Autodesk Inventor part; units mm, degrees
(part 3 of 5)
  arc A1149 (8.6341, 10.3239) -> (7.2074, 10.3304) centre (7.8644, -2.208) ccw
  arc A1150 (10.0591, 10.155) -> (8.6341, 10.3239) centre (7.8573, -2.3245) ccw
  arc A1151 (11.2931, 9.8332) -> (10.0591, 10.155) centre (8.6807, 2.3424) ccw
  arc A1152 (-14.2689, 7.2702) -> (-15.0029, 6.7254) centre (-13.5906, 5.5896) ccw
  arc A1153 (-15.0029, 6.7254) -> (-15.3966, 5.8804) centre (-13.4832, 5.5032) ccw
  arc A1154 (-15.3966, 5.8804) -> (-15.5635, 4.3135) centre (-6.6517, 4.1565) ccw
  arc A1155 (-15.5635, 4.3135) -> (-15.5968, 0.5339) centre (198.9705, 0.534) ccw
  arc A1156 (-15.5968, 0.5339) -> (-15.5855, -2.9927) centre (534.7574, 0.5336) ccw
  arc A1157 (-15.5855, -2.9927) -> (-15.5199, -4.2476) centre (-1.8593, -2.9048) ccw
  arc A1158 (-15.5199, -4.2476) -> (-15.3495, -4.9618) centre (-12.8301, -3.9832) ccw
  arc A1159 (-15.3495, -4.9618) -> (-14.9991, -5.5461) centre (-13.4693, -4.2315) ccw
  arc A1160 (-14.9991, -5.5461) -> (-14.5333, -5.9588) centre (-13.256, -4.0482) ccw
  arc A1161 (-14.5333, -5.9588) -> (-14.0306, -6.1641) centre (-13.7802, -4.8324) ccw
  arc A1162 (-14.0306, -6.1641) -> (-13.1923, -6.2566) centre (-13.0028, -0.6964) ccw
  arc A1163 (-13.1923, -6.2566) -> (-10.8659, -6.323) centre (-6.0064, 204.5863) ccw
  arc A1164 (-10.8659, -6.323) -> (-8.1681, -6.35) centre (-8.4856, 96.9906) ccw
  arc A1165 (-8.1681, -6.35) -> (-6.6957, -6.2434) centre (-8.2009, 4.3293) ccw
  arc A1166 (-6.6957, -6.2434) -> (-5.7509, -5.9784) centre (-7.221, -2.5536) ccw
  arc A1167 (-5.7509, -5.9784) -> (-5.034, -5.4928) centre (-6.6553, -3.8715) ccw
  arc A1168 (-5.034, -5.4928) -> (-4.687, -4.9742) centre (-6.1681, -4.3587) ccw
  arc A1169 (-4.687, -4.9742) -> (-4.518, -4.3054) centre (-6.8723, -4.066) ccw
  arc A1170 (-4.518, -4.3054) -> (-4.453, -3.1016) centre (-17.1608, -3.0197) ccw
  arc A1171 (-4.453, -3.1016) -> (-4.442, 0.3284) centre (-536.7191, 0.3287) ccw
  arc A1172 (-4.442, 0.3284) -> (-4.4832, 4.1346) centre (-180.1506, 0.3283) ccw
  arc A1173 (-4.4832, 4.1346) -> (-4.6809, 5.7903) centre (-13.0751, 3.9485) ccw
  arc A1174 (-4.6809, 5.7903) -> (-5.1333, 6.6851) centre (-6.6435, 5.3596) ccw
  arc A1175 (-5.1333, 6.6851) -> (-5.9587, 7.2413) centre (-6.6019, 5.3961) ccw
  arc A1176 (-5.9587, 7.2413) -> (-7.0837, 7.4475) centre (-7.1851, 3.7233) ccw
  arc A1177 (-7.0837, 7.4475) -> (-10.1664, 7.4949) centre (-10.6188, -122.3153) ccw
  arc A1178 (-10.1664, 7.4949) -> (-13.2748, 7.4725) centre (-10.6734, -137.9503) ccw
  arc A1179 (-13.2748, 7.4725) -> (-14.2689, 7.2702) centre (-13.2249, 4.6832) ccw
  arc A1180 (-14.7169, 5.5669) -> (-14.1838, 6.0865) centre (-34.7338, 26.6365) ccw
  arc A1181 (-14.9423, 5.4172) -> (-14.7169, 5.5669) centre (-15.2572, 6.1357) ccw
  arc A1182 (-15.0561, 5.4626) -> (-14.9423, 5.4172) centre (-14.9769, 5.496) ccw
  arc A1183 (-15.101, 5.6846) -> (-15.0561, 5.4626) centre (-14.5294, 5.6846) ccw
  arc A1184 (-15.0074, 6.0856) -> (-15.101, 5.6846) centre (-14.1956, 5.6846) ccw
  arc A1185 (-14.73, 6.4972) -> (-15.0074, 6.0856) centre (-13.3432, 5.2635) ccw
  arc A1186 (-14.3269, 6.8498) -> (-14.73, 6.4972) centre (-13.1262, 5.0705) ccw
  arc A1187 (-13.8616, 7.0779) -> (-14.3269, 6.8498) centre (-13.2722, 5.2869) ccw
  arc A1188 (-13.5072, 7.1356) -> (-13.8616, 7.0779) centre (-13.5016, 5.9839) ccw
  arc A1189 (-13.4174, 7.0127) -> (-13.5072, 7.1356) centre (-13.5067, 7.0417) ccw
  arc A1190 (-13.6008, 6.6974) -> (-13.4174, 7.0127) centre (-14.2405, 7.2802) ccw
  arc A1191 (-14.1838, 6.0865) -> (-13.6008, 6.6974) centre (-27.0342, 18.9369) ccw
  arc A1192 (-5.369, 6.261) -> (-5.3902, 6.5814) centre (-5.5632, 6.409) ccw
  arc A1193 (-6.1138, 5.3522) -> (-5.369, 6.261) centre (-18.7203, 16.4429) ccw
  arc A1194 (-7.4344, 3.9305) -> (-6.1138, 5.3522) centre (-33.0415, 29.0421) ccw
  arc A1195 (-10.0244, 1.3139) -> (-7.4344, 3.9305) centre (-290.0893, 281.1159) ccw
  arc A1196 (-11.9319, -0.585) -> (-10.0244, 1.3139) centre (-356.2197, 347.1842) ccw
  arc A1197 (-13.5616, -2.1839) -> (-11.9319, -0.585) centre (-190.9648, 180.2579) ccw
  arc A1198 (-15.0178, -3.5983) -> (-13.5616, -2.1839) centre (-1246.2884, 1265.5516) ccw
  arc A1199 (-15.1177, -3.6388) -> (-15.0178, -3.5983) centre (-15.1177, -3.4953) ccw
  arc A1200 (-15.1687, -3.5954) -> (-15.1177, -3.6388) centre (-15.1177, -3.5871) ccw
  arc A1201 (-15.1891, -3.4021) -> (-15.1687, -3.5954) centre (-13.4719, -3.3194) ccw
  arc A1202 (-15.1869, -3.1421) -> (-15.1891, -3.4021) centre (-12.8846, -3.2911) ccw
  arc A1203 (-15.1565, -2.8332) -> (-15.1869, -3.1421) centre (-10.5477, -3.4424) ccw
  arc A1204 (-14.9222, -2.233) -> (-15.1565, -2.8332) centre (-13.8179, -3.0101) ccw
  arc A1205 (-14.2117, -1.3211) -> (-14.9222, -2.233) centre (-5.195, -9.0783) ccw
  arc A1206 (-12.9707, 0.0372) -> (-14.2117, -1.3211) centre (9.1494, -21.4189) ccw
  arc A1207 (-10.6781, 2.3724) -> (-12.9707, 0.0372) centre (182.1892, -189.2648) ccw
  arc A1208 (-10.6781, 2.3724) -> (-9.019, 4.0601) centre (-168.3412, 159.0297) ccw
  arc A1209 (-9.019, 4.0601) -> (-7.6634, 5.4799) centre (-84.9047, 77.8727) ccw
  arc A1210 (-7.6634, 5.4799) -> (-6.5236, 6.7019) centre (-257.9199, 240.0277) ccw
  arc A1211 (-6.5236, 6.7019) -> (-6.5544, 6.7724) centre (-6.5544, 6.7304) ccw
  arc A1212 (-6.5544, 6.7724) -> (-6.7207, 6.7067) centre (-6.5544, 6.5289) ccw
  arc A1213 (-6.7207, 6.7067) -> (-7.9294, 5.5709) centre (238.0969, -255.0416) ccw
  arc A1214 (-7.9294, 5.5709) -> (-9.3033, 4.2502) centre (64.3345, -70.9771) ccw
  arc A1215 (-9.3033, 4.2502) -> (-10.887, 2.6823) centre (127.8746, -135.8883) ccw
  arc A1216 (-12.4629, 1.1142) -> (-10.887, 2.6823) centre (-257.9204, 249.3758) ccw
  arc A1217 (-13.8124, -0.2064) -> (-12.4629, 1.1142) centre (-140.6508, 130.7665) ccw
  arc A1218 (-15.0152, -1.3694) -> (-13.8124, -0.2064) centre (-777.5444, 788.4217) ccw
  arc A1219 (-15.1104, -1.4078) -> (-15.0152, -1.3694) centre (-15.1104, -1.2708) ccw
  arc A1220 (-15.1598, -1.3649) -> (-15.1104, -1.4078) centre (-15.1104, -1.3579) ccw
  arc A1221 (-15.1793, -1.1574) -> (-15.1598, -1.3649) centre (-12.9724, -1.0553) ccw
  arc A1222 (-15.178, -0.8822) -> (-15.1793, -1.1574) centre (-12.4811, -1.0326) ccw
  arc A1223 (-15.1498, -0.5554) -> (-15.178, -0.8822) centre (-9.7652, -1.184) ccw
  arc A1224 (-14.9553, 0.0294) -> (-15.1498, -0.5554) centre (-13.6453, -0.731) ccw
  arc A1225 (-14.4687, 0.7308) -> (-14.9553, 0.0294) centre (-10.3735, -2.6302) ccw
  arc A1226 (-13.5735, 1.7298) -> (-14.4687, 0.7308) centre (-2.5197, -9.0758) ccw
  arc A1227 (-11.8574, 3.4563) -> (-13.5735, 1.7298) centre (90.964, -100.4609) ccw
  arc A1228 (-11.8574, 3.4563) -> (-10.6423, 4.6769) centre (-91.9133, 84.3654) ccw
  arc A1229 (-10.6423, 4.6769) -> (-9.64, 5.7252) centre (-51.7109, 44.9459) ccw
  arc A1230 (-9.64, 5.7252) -> (-8.7905, 6.6422) centre (-153.1351, 139.4989) ccw
  arc A1231 (-8.7905, 6.6422) -> (-8.7926, 6.7438) centre (-8.8445, 6.6919) ccw
  arc A1232 (-8.7926, 6.7438) -> (-8.8943, 6.7463) centre (-8.8448, 6.6916) ccw
  arc A1233 (-8.8943, 6.7463) -> (-9.7737, 5.9459) centre (105.081, -119.365) ccw
  arc A1234 (-9.7737, 5.9459) -> (-10.7808, 4.998) centre (25.5758, -32.6218) ccw
  arc A1235 (-10.7808, 4.998) -> (-11.9525, 3.8475) centre (61.1169, -69.3977) ccw
  arc A1236 (-13.1243, 2.6881) -> (-11.9525, 3.8475) centre (-154.213, 146.4505) ccw
  arc A1237 (-14.1326, 1.7116) -> (-13.1243, 2.6881) centre (-87.5839, 78.5589) ccw
  arc A1238 (-15.0266, 0.8592) -> (-14.1326, 1.7116) centre (-358.2866, 361.7781) ccw
  arc A1239 (-15.1168, 0.8231) -> (-15.0266, 0.8592) centre (-15.1168, 0.954) ccw
  arc A1240 (-15.164, 0.8649) -> (-15.1168, 0.8231) centre (-15.1168, 0.8707) ccw
  arc A1241 (-15.1808, 1.077) -> (-15.164, 0.8649) centre (-12.669, 1.169) ccw
  arc A1242 (-15.1776, 1.3559) -> (-15.1808, 1.077) centre (-12.2736, 1.1835) ccw
  arc A1243 (-15.1485, 1.6872) -> (-15.1776, 1.3559) centre (-9.3449, 1.0097) ccw
  arc A1244 (-14.9951, 2.2222) -> (-15.1485, 1.6872) centre (-13.445, 1.4884) ccw
  arc A1245 (-14.6569, 2.7815) -> (-14.9951, 2.2222) centre (-12.0877, 0.8459) ccw
  arc A1246 (-14.0493, 3.4933) -> (-14.6569, 2.7815) centre (-8.5071, -1.8518) ccw
  arc A1247 (-12.9686, 4.5806) -> (-14.0493, 3.4933) centre (22.4806, -31.7374) ccw
  arc A1248 (-12.9686, 4.5806) -> (-12.1808, 5.368) centre (-45.7482, 38.1635) ccw
  arc A1249 (-12.1808, 5.368) -> (-11.5385, 6.0519) centre (-29.1598, 21.9566) ccw
  arc A1250 (-11.5385, 6.0519) -> (-11.0163, 6.6395) centre (-49.2283, 40.0701) ccw
  arc A1251 (-11.0163, 6.6395) -> (-11.0197, 6.7398) centre (-11.0716, 6.6879) ccw
  arc A1252 (-11.0197, 6.7398) -> (-11.1204, 6.7441) centre (-11.0724, 6.6871) ccw
  arc A1253 (-11.1204, 6.7441) -> (-11.6919, 6.2547) centre (17.8083, -27.6153) ccw
  arc A1254 (-11.6919, 6.2547) -> (-12.3585, 5.6496) centre (2.6791, -10.245) ccw
  arc A1255 (-12.3585, 5.6496) -> (-13.1254, 4.9058) centre (17.2995, -25.6985) ccw
  line L70 (-13.1254, 4.9058) -> (-15.101, 2.9418)
  line L71 (-15.101, 2.9418) -> (-15.101, 3.8604)
  arc A1256 (-15.0485, 4.3869) -> (-15.101, 3.8604) centre (-12.434, 3.8604) ccw
  arc A1257 (-14.8904, 4.8048) -> (-15.0485, 4.3869) centre (-13.698, 4.115) ccw
  arc A1258 (-14.5681, 5.2353) -> (-14.8904, 4.8048) centre (-12.9172, 3.6633) ccw
  arc A1259 (-13.9571, 5.8377) -> (-14.5681, 5.2353) centre (-4.7269, -4.1359) ccw
  arc A1260 (-13.4501, 6.2649) -> (-13.9571, 5.8377) centre (-9.1213, 0.6123) ccw
  arc A1261 (-12.9184, 6.6311) -> (-13.4501, 6.2649) centre (-9.5568, 1.1811) ccw
  arc A1262 (-12.4232, 6.9008) -> (-12.9184, 6.6311) centre (-10.167, 2.1703) ccw
  arc A1263 (-12.0399, 7.0202) -> (-12.4232, 6.9008) centre (-11.817, 5.6299) ccw
  arc A1264 (-10.6511, 7.1146) -> (-12.0399, 7.0202) centre (-10.8287, -0.537) ccw
  arc A1265 (-8.3195, 7.0107) -> (-10.6511, 7.1146) centre (-11.9196, -47.5415) ccw
  arc A1266 (-5.9123, 6.8255) -> (-8.3195, 7.0107) centre (-15.6325, -103.8039) ccw
  arc A1267 (-5.3902, 6.5814) -> (-5.9123, 6.8255) centre (-5.9859, 5.9877) ccw
  arc A1268 (-11.5429, -2.4135) -> (-9.689, -0.5817) centre (-151.916, 141.5052) ccw
  arc A1269 (-13.1444, -3.943) -> (-11.5429, -2.4135) centre (-85.0076, 72.9068) ccw
  arc A1270 (-14.555, -5.2556) -> (-13.1444, -3.943) centre (-278.0551, 279.3503) ccw
  arc A1271 (-14.7274, -5.2932) -> (-14.555, -5.2556) centre (-14.6731, -5.128) ccw
  arc A1272 (-14.8283, -5.2275) -> (-14.7274, -5.2932) centre (-14.6542, -5.0704) ccw
  arc A1273 (-14.9247, -5.0944) -> (-14.8283, -5.2275) centre (-14.2593, -4.7138) ccw
  arc A1274 (-15.0027, -4.9212) -> (-14.9247, -5.0944) centre (-14.0688, -4.6049) ccw
  arc A1275 (-15.0486, -4.7317) -> (-15.0027, -4.9212) centre (-13.9673, -4.5705) ccw
  arc A1276 (-14.9401, -4.3504) -> (-15.0486, -4.7317) centre (-14.5734, -4.6608) ccw
  arc A1277 (-13.9274, -3.1917) -> (-14.9401, -4.3504) centre (22.1213, -35.7196) ccw
  arc A1278 (-12.4307, -1.5992) -> (-13.9274, -3.1917) centre (26.1037, -39.313) ccw
  arc A1279 (-10.0909, 0.7626) -> (-12.4307, -1.5992) centre (182.391, -192.2721) ccw
  arc A1280 (-6.8029, 4.0259) -> (-10.0909, 0.7626) centre (688.2331, -699.5646) ccw
  arc A1281 (-5.7215, 5.0044) -> (-6.8029, 4.0259) centre (4.9025, -7.8236) ccw
  arc A1282 (-5.2387, 5.2053) -> (-5.7215, 5.0044) centre (-5.152, 4.3167) ccw
  arc A1283 (-4.9809, 4.9946) -> (-5.2387, 5.2053) centre (-5.2158, 4.9704) ccw
  arc A1284 (-5.1077, 4.3788) -> (-4.9809, 4.9946) centre (-6.0196, 4.8875) ccw
  arc A1285 (-5.6506, 3.5937) -> (-5.1077, 4.3788) centre (-9.4491, 6.8007) ccw
  arc A1286 (-6.807, 2.3253) -> (-5.6506, 3.5937) centre (-22.8922, 18.1506) ccw
  arc A1287 (-9.689, -0.5817) -> (-6.807, 2.3253) centre (-388.1467, 377.5026) ccw
  arc A1288 (-11.1643, -4.2674) -> (-8.8203, -1.944) centre (-236.5359, 225.4382) ccw
  arc A1289 (-12.2567, -5.2477) -> (-11.1643, -4.2674) centre (-22.7028, 7.4931) ccw
  arc A1290 (-12.9748, -5.7175) -> (-12.2567, -5.2477) centre (-14.7932, -2.154) ccw
  arc A1291 (-13.6083, -5.8698) -> (-12.9748, -5.7175) centre (-13.6083, -4.4759) ccw
  arc A1292 (-13.8587, -5.6594) -> (-13.6083, -5.8698) centre (-13.6083, -5.6156) ccw
  arc A1293 (-13.7543, -5.259) -> (-13.8587, -5.6594) centre (-13.368, -5.5736) ccw
  arc A1294 (-12.8767, -4.2816) -> (-13.7543, -5.259) centre (-3.2069, -13.8466) ccw
  arc A1295 (-9.769, -1.1543) -> (-12.8767, -4.2816) centre (670.3181, -680.0673) ccw
  arc A1296 (-6.6738, 1.9312) -> (-9.769, -1.1543) centre (626.6559, -636.4816) ccw
  arc A1297 (-5.6713, 2.8358) -> (-6.6738, 1.9312) centre (3.3784, -8.2017) ccw
  arc A1298 (-5.2271, 2.9942) -> (-5.6713, 2.8358) centre (-5.2284, 2.2957) ccw
  arc A1299 (-4.981, 2.7715) -> (-5.2271, 2.9942) centre (-5.2276, 2.7463) ccw
  arc A1300 (-5.0849, 2.1811) -> (-4.981, 2.7715) centre (-6.0751, 2.6597) ccw
  arc A1301 (-5.5218, 1.4946) -> (-5.0849, 2.1811) centre (-8.235, 3.7036) ccw
  arc A1302 (-6.4749, 0.4278) -> (-5.5218, 1.4946) centre (-17.6327, 11.3551) ccw
  arc A1303 (-8.8203, -1.944) -> (-6.4749, 0.4278) centre (-252.0588, 240.9382) ccw
  arc A1304 (-4.9861, -3.5076) -> (-4.9712, -1.7177) centre (-109.4566, -1.7426) ccw
  arc A1305 (-5.0546, -4.3559) -> (-4.9861, -3.5076) centre (-11.6752, -3.3946) ccw
  arc A1306 (-5.2075, -4.8827) -> (-5.0546, -4.3559) centre (-7.0219, -4.0703) ccw
  arc A1307 (-5.4931, -5.312) -> (-5.2075, -4.8827) centre (-6.6319, -4.2449) ccw
  arc A1308 (-5.7778, -5.5571) -> (-5.4931, -5.312) centre (-6.7749, -4.1109) ccw
  arc A1309 (-6.1037, -5.7315) -> (-5.7778, -5.5571) centre (-6.7139, -4.1994) ccw
  arc A1310 (-6.4748, -5.8351) -> (-6.1037, -5.7315) centre (-6.772, -4.0536) ccw
  arc A1311 (-6.8936, -5.8698) -> (-6.4748, -5.8351) centre (-6.8936, -3.3244) ccw
  line L72 (-6.8936, -5.8698) -> (-7.7715, -5.8698)
  line L73 (-7.7715, -5.8698) -> (-6.4785, -4.5606)
  arc A1312 (-6.4785, -4.5606) -> (-5.9832, -4.042) centre (-21.8725, 10.6422) ccw
  arc A1313 (-5.9832, -4.042) -> (-5.5654, -3.5675) centre (-15.6012, 4.8466) ccw
  arc A1314 (-5.5654, -3.5675) -> (-5.235, -3.1609) centre (-18.6733, 7.4222) ccw
  arc A1315 (-5.235, -3.1609) -> (-5.1856, -3.0184) centre (-5.4159, -3.0184) ccw
  arc A1316 (-5.1856, -3.0184) -> (-5.2482, -2.9874) centre (-5.2246, -3.0184) ccw
  arc A1317 (-5.2482, -2.9874) -> (-5.6407, -3.2991) centre (2.2216, -12.7978) ccw
  arc A1318 (-5.6407, -3.2991) -> (-6.1404, -3.7359) centre (2.195, -12.7657) ccw
  arc A1319 (-6.1404, -3.7359) -> (-6.7349, -4.3008) centre (13.1199, -24.6008) ccw
  arc A1320 (-7.4945, -5.0061) -> (-6.7349, -4.3008) centre (-20.6865, 9.9637) ccw
  arc A1321 (-8.1102, -5.4868) -> (-7.4945, -5.0061) centre (-11.8413, -0.0736) ccw
  arc A1322 (-8.6313, -5.7878) -> (-8.1102, -5.4868) centre (-10.2556, -2.3741) ccw
  arc A1323 (-9.0898, -5.9239) -> (-8.6313, -5.7878) centre (-9.2946, -4.3938) ccw
  arc A1324 (-9.3987, -5.9546) -> (-9.0898, -5.9239) centre (-9.696, -1.3946) ccw
  arc A1325 (-9.6588, -5.9567) -> (-9.3987, -5.9546) centre (-9.5462, -3.6923) ccw
  arc A1326 (-9.8515, -5.9358) -> (-9.6588, -5.9567) centre (-9.5762, -4.295) ccw
  arc A1327 (-9.8954, -5.8839) -> (-9.8515, -5.9358) centre (-9.8428, -5.8839) ccw
  arc A1328 (-9.8564, -5.785) -> (-9.8954, -5.8839) centre (-9.7507, -5.8839) ccw
  arc A1329 (-9.2037, -5.0906) -> (-9.8564, -5.785) centre (130.4768, -137.0342) ccw
  arc A1330 (-8.4432, -4.3005) -> (-9.2037, -5.0906) centre (33.2795, -45.2206) ccw
  arc A1331 (-7.5405, -3.3909) -> (-8.4432, -4.3005) centre (69.1214, -80.3729) ccw
  arc A1332 (-7.5405, -3.3909) -> (-6.638, -2.4741) centre (-53.3898, 42.6497) ccw
  arc A1333 (-6.638, -2.4741) -> (-5.8774, -1.6617) centre (-32.9016, 22.8749) ccw
  arc A1334 (-5.8774, -1.6617) -> (-5.2464, -0.9577) centre (-60.4698, 47.9053) ccw
  arc A1335 (-5.2464, -0.9577) -> (-5.1856, -0.7972) centre (-5.4278, -0.7972) ccw
  arc A1336 (-5.1856, -0.7972) -> (-5.2548, -0.7657) centre (-5.2274, -0.7972) ccw
  arc A1337 (-5.2548, -0.7657) -> (-5.9684, -1.3956) centre (38.7824, -51.3747) ccw
  arc A1338 (-5.9684, -1.3956) -> (-6.8281, -2.1903) centre (18.6502, -28.8905) ccw
  arc A1339 (-6.8281, -2.1903) -> (-7.8504, -3.1832) centre (48.7205, -60.4029) ccw
  arc A1340 (-9.2202, -4.5061) -> (-7.8504, -3.1832) centre (-64.9801, 54.6016) ccw
  arc A1341 (-10.1256, -5.2882) -> (-9.2202, -4.5061) centre (-18.5892, 5.4254) ccw
  arc A1342 (-10.7924, -5.7434) -> (-10.1256, -5.2882) centre (-13.7225, -0.7351) ccw
  arc A1343 (-11.3208, -5.9248) -> (-10.7924, -5.7434) centre (-11.5071, -4.5219) ccw
  arc A1344 (-11.6297, -5.9557) -> (-11.3208, -5.9248) centre (-11.957, -1.1342) ccw
  arc A1345 (-11.8897, -5.9593) -> (-11.6297, -5.9557) centre (-11.792, -3.5647) ccw
  arc A1346 (-12.084, -5.941) -> (-11.8897, -5.9593) centre (-11.8145, -4.1167) ccw
  arc A1347 (-12.1264, -5.8919) -> (-12.084, -5.941) centre (-12.0768, -5.8919) ccw
  arc A1348 (-12.0627, -5.7363) -> (-12.1264, -5.8919) centre (-11.9047, -5.8919) ccw
  arc A1349 (-8.6188, -2.2402) -> (-12.0627, -5.7363) centre (7273.2468, -7178.6542) ccw
  arc A1350 (-5.1724, 1.2552) -> (-8.6188, -2.2402) centre (7336.2909, -7240.7819) ccw
  arc A1351 (-5.02, 1.3189) -> (-5.1724, 1.2552) centre (-5.02, 1.1048) ccw
  arc A1352 (-5.0003, 1.2995) -> (-5.02, 1.3189) centre (-5.02, 1.2992) ccw
  arc A1353 (-4.9858, 0.4269) -> (-5.0003, 1.2995) centre (-888.2077, -13.7685) ccw
  arc A1354 (-4.9749, -0.5533) -> (-4.9858, 0.4269) centre (-103.9909, -1.1645) ccw
  arc A1355 (-4.9712, -1.7177) -> (-4.9749, -0.5533) centre (-201.1281, -1.7643) ccw
  arc A1356 (-47.5872, 6.4838) -> (-47.7919, 6.3363) centre (-38.3913, -6.4958) ccw
  arc A1357 (-47.7919, 6.3363) -> (-47.8023, 6.3017) centre (-47.7742, 6.3122) ccw
  arc A1358 (-47.8023, 6.3017) -> (-47.7727, 6.287) centre (-47.7796, 6.3101) ccw
  arc A1359 (-47.7727, 6.287) -> (-47.5404, 6.3585) centre (-51.7296, 19.5602) ccw
  arc A1360 (-47.3446, 6.3797) -> (-47.5404, 6.3585) centre (-47.39, 5.8845) ccw
  arc A1361 (-47.088, 6.333) -> (-47.3446, 6.3797) centre (-47.4787, 4.9144) ccw
  arc A1362 (-46.816, 6.2331) -> (-47.088, 6.333) centre (-47.5516, 4.6499) ccw
  arc A1363 (-46.5697, 6.0911) -> (-46.816, 6.2331) centre (-47.4973, 4.7667) ccw
  arc A1364 (-46.5697, 6.0911) -> (-46.3623, 5.9563) centre (-44.5142, 9.0258) ccw
  arc A1365 (-46.3623, 5.9563) -> (-46.223, 5.8964) centre (-46.0747, 6.434) ccw
  arc A1366 (-46.223, 5.8964) -> (-46.1771, 5.9196) centre (-46.2128, 5.9333) ccw
  arc A1367 (-46.1771, 5.9196) -> (-46.1832, 5.9845) centre (-46.2457, 5.9459) ccw
  arc A1368 (-46.1832, 5.9845) -> (-46.4751, 6.3144) centre (-47.2857, 5.3031) ccw
  arc A1369 (-46.4751, 6.3144) -> (-46.8627, 6.5306) centre (-47.31, 5.2728) ccw
  arc A1370 (-46.8627, 6.5306) -> (-47.2615, 6.5931) centre (-47.2279, 5.5037) ccw
  arc A1371 (-47.2615, 6.5931) -> (-47.5872, 6.4838) centre (-47.2431, 5.9981) ccw
  arc A1372 (-48.0789, 4.9627) -> (-47.7011, 4.6858) centre (-47.4249, 5.4589) ccw
  arc A1373 (-47.7011, 4.6858) -> (-47.1514, 4.5938) centre (-47.1694, 6.174) ccw
  arc A1374 (-47.1514, 4.5938) -> (-46.6597, 4.7) centre (-47.1657, 5.8505) ccw
  arc A1375 (-46.6597, 4.7) -> (-46.4341, 4.9814) centre (-46.8168, 5.0571) ccw
  arc A1376 (-46.4341, 4.9814) -> (-46.415, 5.0949) centre (-48.4188, 5.3738) ccw
  arc A1377 (-46.415, 5.0949) -> (-46.427, 5.13) centre (-46.4557, 5.1006) ccw
  arc A1378 (-46.427, 5.13) -> (-46.4514, 5.1269) centre (-46.438, 5.1187) ccw
  arc A1379 (-46.4514, 5.1269) -> (-46.4976, 5.0434) centre (-45.5437, 4.5703) ccw
  arc A1380 (-46.736, 4.8493) -> (-46.4976, 5.0434) centre (-46.8301, 5.2083) ccw
  arc A1381 (-47.1922, 4.7987) -> (-46.736, 4.8493) centre (-47.1363, 6.3761) ccw
  arc A1382 (-47.6925, 4.8847) -> (-47.1922, 4.7987) centre (-47.1253, 6.6865) ccw
  arc A1383 (-48.0701, 5.0991) -> (-47.6925, 4.8847) centre (-47.3821, 5.8707) ccw
  arc A1384 (-48.0701, 5.0991) -> (-48.2761, 5.2809) centre (-65.2264, -14.1402) ccw
  arc A1385 (-48.2761, 5.2809) -> (-48.2944, 5.2732) centre (-48.2833, 5.2725) ccw
  arc A1386 (-48.2944, 5.2732) -> (-48.2822, 5.2323) centre (-48.2328, 5.2693) ccw
  arc A1387 (-48.2822, 5.2323) -> (-48.0789, 4.9627) centre (-3.2497, 38.9768) ccw
  arc A1388 (-54.9842, 2.087) -> (-55.6668, 0.9823) centre (-53.2977, 0.2817) ccw
  arc A1389 (-55.6668, 0.9823) -> (-55.6108, -0.2103) centre (-53.9229, 0.4666) ccw
  arc A1390 (-55.6108, -0.2103) -> (-54.8228, -1.1293) centre (-53.8639, 0.4902) ccw
  arc A1391 (-54.8228, -1.1293) -> (-53.5471, -1.4967) centre (-53.4779, 1.142) ccw
  arc A1392 (-53.5471, -1.4967) -> (-52.9687, -1.4805) centre (-53.4075, 3.8295) ccw
  arc A1393 (-52.9687, -1.4805) -> (-52.5723, -1.387) centre (-53.0816, -0.114) ccw
  arc A1394 (-52.5723, -1.387) -> (-52.2428, -1.1875) centre (-53.0105, -0.2916) ccw
  arc A1395 (-52.2428, -1.1875) -> (-51.8873, -0.8327) centre (-54.3957, 1.3249) ccw
  arc A1396 (-51.8873, -0.8327) -> (-51.3873, 0.05) centre (-53.8722, 0.8746) ccw
  arc A1397 (-51.3873, 0.05) -> (-51.3289, 0.9689) centre (-53.107, 0.6207) ccw
  arc A1398 (-51.3289, 0.9689) -> (-51.7297, 1.7992) centre (-53.1132, 0.6195) ccw
  arc A1399 (-51.7297, 1.7992) -> (-52.5266, 2.4318) centre (-53.7404, 0.0846) ccw
  arc A1400 (-52.5266, 2.4318) -> (-53.246, 2.7227) centre (-54.4468, -1.2814) ccw
  arc A1401 (-53.246, 2.7227) -> (-53.8229, 2.7667) centre (-53.6349, 1.426) ccw
  arc A1402 (-53.8229, 2.7667) -> (-54.3672, 2.5657) centre (-53.6335, 1.4164) ccw
  arc A1403 (-54.3672, 2.5657) -> (-54.9842, 2.087) centre (-52.0702, -1.0324) ccw
  arc A1404 (-51.9454, 1.3028) -> (-52.2837, 1.8147) centre (-53.3677, 0.7307) ccw
  arc A1405 (-51.8069, 0.6651) -> (-51.9454, 1.3028) centre (-53.7496, 0.577) ccw
  arc A1406 (-51.8856, -0.0049) -> (-51.8069, 0.6651) centre (-53.8932, 0.5705) ccw
  arc A1407 (-52.1738, -0.609) -> (-51.8856, -0.0049) centre (-53.8334, 0.5534) ccw
  arc A1408 (-52.6738, -1.0129) -> (-52.1738, -0.609) centre (-53.1252, 0.0574) ccw
  arc A1409 (-53.3968, -1.1672) -> (-52.6738, -1.0129) centre (-53.4388, 0.8008) ccw
  arc A1410 (-54.1575, -1.0453) -> (-53.3968, -1.1672) centre (-53.4426, 0.9823) ccw
  arc A1411 (-54.7625, -0.6642) -> (-54.1575, -1.0453) centre (-53.6205, 0.4779) ccw
  arc A1412 (-55.2241, 0.217) -> (-54.7625, -0.6642) centre (-53.5836, 0.5148) ccw
  arc A1413 (-55.1151, 1.2255) -> (-55.2241, 0.217) centre (-53.4623, 0.5368) ccw
  arc A1414 (-54.4754, 2.0144) -> (-55.1151, 1.2255) centre (-53.4567, 0.5345) ccw
  arc A1415 (-53.5231, 2.3104) -> (-54.4754, 2.0144) centre (-53.5231, 0.6309) ccw
  arc A1416 (-53.2004, 2.2743) -> (-53.5231, 2.3104) centre (-53.5231, 0.8503) ccw
  arc A1417 (-52.8518, 2.1658) -> (-53.2004, 2.2743) centre (-53.7128, 0.0131) ccw
  arc A1418 (-52.5288, 2.0058) -> (-52.8518, 2.1658) centre (-53.695, 0.0578) ccw
  arc A1419 (-52.2837, 1.8147) -> (-52.5288, 2.0058) centre (-53.1795, 0.9189) ccw
  arc A1420 (-48.0201, -3.6884) -> (-48.1327, -3.8305) centre (-47.4621, -4.2464) ccw
  arc A1421 (-48.1327, -3.8305) -> (-48.2252, -4.0113) centre (-47.0822, -4.4819) ccw
  arc A1422 (-48.2252, -4.0113) -> (-48.2855, -4.2012) centre (-47.1181, -4.4672) ccw
  arc A1423 (-48.2855, -4.2012) -> (-48.3008, -4.37) centre (-47.666, -4.3423) ccw
  arc A1424 (-48.3008, -4.37) -> (-48.2766, -4.5038) centre (-47.7965, -4.348) ccw
  arc A1425 (-48.2766, -4.5038) -> (-48.223, -4.5245) centre (-48.2414, -4.4924) ccw
  arc A1426 (-48.223, -4.5245) -> (-48.1426, -4.4432) centre (-48.3295, -4.3385) ccw
  arc A1427 (-48.1426, -4.4432) -> (-48.0209, -4.2099) centre (-51.9333, -2.3195) ccw
  arc A1428 (-47.8586, -3.9745) -> (-48.0209, -4.2099) centre (-47.1804, -4.616) ccw
  arc A1429 (-47.6236, -3.783) -> (-47.8586, -3.9745) centre (-47.005, -4.7819) ccw
  arc A1430 (-47.3272, -3.645) -> (-47.6236, -3.783) centre (-46.8972, -4.9559) ccw
  arc A1431 (-46.9842, -3.5678) -> (-47.3272, -3.645) centre (-46.7541, -5.3923) ccw
  line L74 (-46.9842, -3.5678) -> (-46.2105, -3.4702)
  line L75 (-46.2105, -3.4702) -> (-46.9666, -3.4306)
  arc A1432 (-46.9666, -3.4306) -> (-47.2778, -3.4374) centre (-47.0766, -5.5275) ccw
  arc A1433 (-47.2778, -3.4374) -> (-47.5879, -3.4899) centre (-47.0683, -5.6132) ccw
  arc A1434 (-47.5879, -3.4899) -> (-47.8531, -3.5768) centre (-47.1538, -5.264) ccw
  arc A1435 (-47.8531, -3.5768) -> (-48.0201, -3.6884) centre (-47.656, -4.0525) ccw
  arc A1436 (-46.6917, -5.01) -> (-46.8592, -5.1502) centre (-45.3579, -6.7735) ccw
  arc A1437 (-46.8592, -5.1502) -> (-46.9537, -5.2671) centre (-46.5039, -5.5344) ccw
  arc A1438 (-46.9537, -5.2671) -> (-46.9597, -5.3384) centre (-46.8832, -5.309) ccw
  arc A1439 (-46.9597, -5.3384) -> (-46.908, -5.374) centre (-46.908, -5.3185) ccw
  arc A1440 (-46.908, -5.374) -> (-46.7846, -5.3481) centre (-46.908, -5.0676) ccw
  arc A1441 (-46.7846, -5.3481) -> (-46.6302, -5.2648) centre (-47.2239, -4.349) ccw
  arc A1442 (-46.6302, -5.2648) -> (-46.4721, -5.1444) centre (-47.3486, -4.1567) ccw
  arc A1443 (-46.4721, -5.1444) -> (-46.3345, -5.0022) centre (-47.3359, -4.171) ccw
  arc A1444 (-46.3345, -5.0022) -> (-46.1066, -4.7102) centre (-51.1085, -1.0401) ccw
  arc A1445 (-46.1066, -4.7102) -> (-46.1351, -4.6553) centre (-46.1344, -4.6898) ccw
  arc A1446 (-46.1351, -4.6553) -> (-46.2723, -4.7011) centre (-46.1297, -4.8998) ccw
  arc A1447 (-46.2723, -4.7011) -> (-46.6917, -5.01) centre (-34.2808, -21.4187) ccw
  arc A1448 (-48.0696, -5.1261) -> (-47.9091, -5.2181) centre (-47.1309, -3.6735) ccw
  arc A1449 (-47.9091, -5.2181) -> (-47.7342, -5.2958) centre (-47.0192, -3.4519) ccw
  arc A1450 (-47.7342, -5.2958) -> (-47.5707, -5.35) centre (-47.1104, -3.6869) ccw
  arc A1451 (-47.5707, -5.35) -> (-47.4499, -5.3664) centre (-47.4499, -4.9136) ccw
  arc A1452 (-47.4499, -5.3664) -> (-47.3924, -5.3436) centre (-47.4499, -5.2821) ccw
  arc A1453 (-47.3924, -5.3436) -> (-47.3841, -5.2958) centre (-47.4199, -5.3143) ccw
  arc A1454 (-47.3841, -5.2958) -> (-47.4464, -5.2189) centre (-47.6003, -5.4073) ccw
  arc A1455 (-47.4464, -5.2189) -> (-47.5739, -5.1261) centre (-48.3441, -6.318) ccw
  arc A1456 (-47.5739, -5.1261) -> (-47.7344, -5.0341) centre (-48.5126, -6.5787) ccw
  arc A1457 (-47.7344, -5.0341) -> (-47.9093, -4.9564) centre (-48.6243, -6.8003) ccw
  arc A1458 (-47.9093, -4.9564) -> (-48.0728, -4.9022) centre (-48.5332, -6.5653) ccw
  arc A1459 (-48.0728, -4.9022) -> (-48.1936, -4.8858) centre (-48.1936, -5.3386) ccw
  arc A1460 (-48.1936, -4.8858) -> (-48.2512, -4.9085) centre (-48.1936, -4.9701) ccw
  arc A1461 (-48.2512, -4.9085) -> (-48.2594, -4.9564) centre (-48.2237, -4.9379) ccw
  arc A1462 (-48.2594, -4.9564) -> (-48.1971, -5.0333) centre (-48.0432, -4.8448) ccw
  arc A1463 (-48.1971, -5.0333) -> (-48.0696, -5.1261) centre (-47.2994, -3.9342) ccw
  arc A1464 (-28.2732, -5.574) -> (-28.5168, -5.8584) centre (-27.8393, -6.1922) ccw
  arc A1465 (-28.5168, -5.8584) -> (-28.6535, -6.2864) centre (-27.1573, -6.5281) ccw
  arc A1466 (-28.6535, -6.2864) -> (-28.7191, -7.0064) centre (-23.4918, -7.1203) ccw
  arc A1467 (-28.7191, -7.0064) -> (-28.7346, -8.43) centre (36.6219, -8.43) ccw
  line L76 (-28.7346, -8.43) -> (-28.7346, -10.9622)
  line L77 (-28.7346, -10.9622) -> (-27.6117, -12.1853)
  line L78 (-27.6117, -12.1853) -> (-26.4888, -13.4084)
  line L79 (-26.4888, -13.4084) -> (-23.1484, -10.075)
  arc A1468 (-21.3525, -8.3073) -> (-23.1484, -10.075) centre (105.8396, -139.3289) ccw
  arc A1469 (-20.3731, -7.432) -> (-21.3525, -8.3073) centre (-10.2474, -19.7467) ccw
  arc A1470 (-19.7489, -6.9923) -> (-20.3731, -7.432) centre (-17.1151, -11.3943) ccw
  arc A1471 (-19.4042, -6.9963) -> (-19.7489, -6.9923) centre (-19.5799, -7.2748) ccw
  arc A1472 (-19.2503, -7.1087) -> (-19.4042, -6.9963) centre (-20.1555, -8.1874) ccw
  arc A1473 (-19.1214, -7.2355) -> (-19.2503, -7.1087) centre (-19.984, -7.983) ccw
  arc A1474 (-19.0328, -7.3579) -> (-19.1214, -7.2355) centre (-19.7766, -7.8033) ccw
  arc A1475 (-19.0086, -7.4529) -> (-19.0328, -7.3579) centre (-19.1797, -7.4459) ccw
  arc A1476 (-19.0648, -7.5881) -> (-19.0086, -7.4529) centre (-19.2205, -7.4442) ccw
  arc A1477 (-19.9429, -8.5337) -> (-19.0648, -7.5881) centre (-217.3375, 175.6569) ccw
  arc A1478 (-20.9654, -9.61) -> (-19.9429, -8.5337) centre (-80.3638, 47.8456) ccw
  arc A1479 (-22.1776, -10.849) -> (-20.9654, -9.61) centre (-130.9902, 96.8162) ccw
  arc A1480 (-24.0448, -12.7158) -> (-22.1776, -10.849) centre (-194.9979, 160.1492) ccw
  arc A1481 (-24.8728, -13.4507) -> (-24.0448, -12.7158) centre (-31.2632, -5.4166) ccw
  arc A1482 (-25.3484, -13.7097) -> (-24.8728, -13.4507) centre (-25.8516, -12.2202) ccw
  arc A1483 (-25.6528, -13.6133) -> (-25.3484, -13.7097) centre (-25.4348, -13.4538) ccw
  arc A1484 (-25.6528, -13.6133) -> (-25.7858, -13.4611) centre (-26.5955, -14.3026) ccw
  arc A1485 (-25.7858, -13.4611) -> (-25.9253, -13.3598) centre (-26.219, -13.9113) ccw
  arc A1486 (-25.9253, -13.3598) -> (-26.0491, -13.3224) centre (-26.0816, -13.6532) ccw
  arc A1487 (-26.0491, -13.3224) -> (-26.1388, -13.3545) centre (-26.06, -13.4333) ccw
  arc A1488 (-26.1388, -13.3545) -> (-26.1413, -13.6754) centre (-25.977, -13.5162) ccw
  arc A1489 (-26.1413, -13.6754) -> (-24.322, -15.5252) centre (95.7981, 104.4298) ccw
  arc A1490 (-24.322, -15.5252) -> (-22.5035, -17.309) centre (62.9595, 71.6366) ccw
  arc A1491 (-22.5035, -17.309) -> (-21.9787, -17.5203) centre (-21.9787, -16.7628) ccw
  arc A1492 (-21.9787, -17.5203) -> (-21.3796, -17.3874) centre (-21.9787, -16.1034) ccw
  arc A1493 (-21.3796, -17.3874) -> (-18.4307, -15.997) centre (-192.0716, 348.4457) ccw
  arc A1494 (-18.4307, -15.997) -> (-15.5918, -14.6227) centre (-127.4533, 212.8237) ccw
  arc A1495 (-15.5918, -14.6227) -> (-14.7911, -14.0958) centre (-17.2888, -11.172) ccw
  arc A1496 (-14.7911, -14.0958) -> (-14.5875, -13.8415) centre (-15.3556, -13.435) ccw
  arc A1497 (-14.5875, -13.8415) -> (-14.4544, -13.4901) centre (-15.9236, -13.1345) ccw
  arc A1498 (-14.4544, -13.4901) -> (-14.3798, -13.0002) centre (-17.2426, -12.8152) ccw
  arc A1499 (-14.3798, -13.0002) -> (-14.3573, -12.3038) centre (-25.1558, -12.3038) ccw
  arc A1500 (-14.3573, -12.3038) -> (-14.4628, -11.1978) centre (-20.2096, -12.3038) ccw
  arc A1501 (-14.4628, -11.1978) -> (-14.7964, -10.4635) centre (-16.1542, -11.5233) ccw
  arc A1502 (-14.7964, -10.4635) -> (-15.5806, -9.65) centre (-19.0746, -13.8029) ccw
  arc A1503 (-15.5806, -9.65) -> (-17.9814, -7.6611) centre (-147.7014, -166.6845) ccw
  line L80 (-17.9814, -7.6611) -> (-20.7378, -5.4126)
  line L81 (-20.7378, -5.4126) -> (-24.2748, -5.3313)
  arc A1504 (-24.2748, -5.3313) -> (-26.0018, -5.3081) centre (-26.3564, -95.9231) ccw
  arc A1505 (-26.0018, -5.3081) -> (-27.1286, -5.34) centre (-26.0702, -22.7818) ccw
  arc A1506 (-27.1286, -5.34) -> (-27.8876, -5.4197) centre (-26.6035, -13.994) ccw
  arc A1507 (-27.8876, -5.4197) -> (-28.2732, -5.574) centre (-27.7536, -6.3142) ccw
  arc A1508 (-27.4301, -7.1648) -> (-26.9995, -6.7373) centre (-43.5695, 9.5249) ccw
  arc A1509 (-27.8177, -7.5252) -> (-27.4301, -7.1648) centre (-36.7939, 2.5183) ccw
  arc A1510 (-28.1514, -7.8172) -> (-27.8177, -7.5252) centre (-42.127, 8.4855) ccw
  arc A1511 (-28.2476, -7.8528) -> (-28.1514, -7.8172) centre (-28.2476, -7.705) ccw
  arc A1512 (-28.3383, -7.7594) -> (-28.2476, -7.8528) centre (-28.2476, -7.7621) ccw
  arc A1513 (-28.3053, -7.1248) -> (-28.3383, -7.7594) centre (-14.261, -8.172) ccw
  arc A1514 (-28.2286, -6.4607) -> (-28.3053, -7.1248) centre (-20.1054, -7.7362) ccw
  arc A1515 (-28.1043, -5.9317) -> (-28.2286, -6.4607) centre (-24.6431, -7.0237) ccw
  arc A1516 (-27.9974, -5.8058) -> (-28.1043, -5.9317) centre (-27.9012, -5.9958) ccw
  arc A1517 (-27.742, -5.7079) -> (-27.9974, -5.8058) centre (-27.3943, -6.997) ccw
  arc A1518 (-27.3867, -5.643) -> (-27.742, -5.7079) centre (-27.1734, -7.8159) ccw
  arc A1519 (-26.9556, -5.6219) -> (-27.3867, -5.643) centre (-26.9556, -10.0338) ccw
  line L82 (-26.9556, -5.6219) -> (-25.9047, -5.6219)
  line L83 (-25.9047, -5.6219) -> (-26.9995, -6.7373)
  arc A1520 (-26.7603, -8.8361) -> (-25.8984, -7.9438) centre (-102.625, 65.2993) ccw
  arc A1521 (-27.5139, -9.5933) -> (-26.7603, -8.8361) centre (-68.6026, 32.0524) ccw
  arc A1522 (-28.173, -10.2399) -> (-27.5139, -9.5933) centre (-140.9676, 105.3981) ccw
  arc A1523 (-28.2853, -10.2987) -> (-28.173, -10.2399) centre (-28.3273, -10.0818) ccw
  arc A1524 (-28.3434, -10.2582) -> (-28.2853, -10.2987) centre (-28.2947, -10.2502) ccw
  arc A1525 (-28.3636, -10.0489) -> (-28.3434, -10.2582) centre (-26.7633, -10.0001) ccw
  arc A1526 (-28.3553, -9.7563) -> (-28.3636, -10.0489) centre (-25.8742, -9.973) ccw
  arc A1527 (-28.3126, -9.4021) -> (-28.3553, -9.7563) centre (-22.929, -10.2303) ccw
  arc A1528 (-28.1729, -8.8974) -> (-28.3126, -9.4021) centre (-26.1032, -9.742) ccw
  arc A1529 (-27.9035, -8.3618) -> (-28.1729, -8.8974) centre (-24.6395, -10.3392) ccw
  arc A1530 (-27.4891, -7.7661) -> (-27.9035, -8.3618) centre (-22.9808, -11.3441) ccw
  arc A1531 (-26.9029, -7.0752) -> (-27.4891, -7.7661) centre (-16.6609, -16.3601) ccw
  arc A1532 (-26.1619, -6.2949) -> (-26.9029, -7.0752) centre (-9.6253, -22.7381) ccw
  arc A1533 (-25.6856, -5.912) -> (-26.1619, -6.2949) centre (-24.2086, -8.2372) ccw
  arc A1534 (-25.2375, -5.7243) -> (-25.6856, -5.912) centre (-24.9125, -7.129) ccw
  arc A1535 (-24.659, -5.6499) -> (-25.2375, -5.7243) centre (-24.5748, -8.5889) ccw
  line L84 (-24.659, -5.6499) -> (-23.682, -5.6219)
  line L85 (-23.682, -5.6219) -> (-25.8984, -7.9438)
  arc A1536 (-26.3562, -10.5347) -> (-24.4561, -8.6534) centre (-214.1373, 181.0275) ccw
  arc A1537 (-27.1092, -11.1826) -> (-26.3562, -10.5347) centre (-31.7158, -5.0672) ccw
  arc A1538 (-27.5566, -11.3736) -> (-27.1092, -11.1826) centre (-27.72, -10.3718) ccw
  arc A1539 (-27.9142, -11.2583) -> (-27.5566, -11.3736) centre (-27.6229, -10.967) ccw
  arc A1540 (-28.0493, -10.9185) -> (-27.9142, -11.2583) centre (-27.5876, -10.9317) ccw
  arc A1541 (-27.9203, -10.5202) -> (-28.0493, -10.9185) centre (-27.3042, -10.9398) ccw
  arc A1542 (-27.4016, -9.8725) -> (-27.9203, -10.5202) centre (-23.4916, -13.5359) ccw
  arc A1543 (-25.873, -8.2606) -> (-27.4016, -9.8725) centre (107.0624, -135.8561) ccw
  arc A1544 (-24.3681, -6.7197) -> (-25.873, -8.2606) centre (63.8859, -94.414) ccw
  arc A1545 (-23.6306, -6.0766) -> (-24.3681, -6.7197) centre (-19.5093, -11.5477) ccw
  arc A1546 (-23.0619, -5.7748) -> (-23.6306, -6.0766) centre (-22.3976, -7.7134) ccw
  arc A1547 (-22.4149, -5.6557) -> (-23.0619, -5.7748) centre (-22.3387, -7.8852) ccw
  line L86 (-22.4149, -5.6557) -> (-21.4246, -5.6219)
  line L87 (-21.4246, -5.6219) -> (-24.4561, -8.6534)
  arc A1548 (-20.3797, -6.4407) -> (-20.4765, -6.0668) centre (-20.7853, -6.3463) ccw
  arc A1549 (-20.6056, -6.9177) -> (-20.3797, -6.4407) centre (-21.5921, -6.1585) ccw
  arc A1550 (-21.3047, -7.7206) -> (-20.6056, -6.9177) centre (-27.5891, -1.5431) ccw
  arc A1551 (-23.2841, -9.7149) -> (-21.3047, -7.7206) centre (-228.0575, 195.5142) ccw
  arc A1552 (-25.3116, -11.7199) -> (-23.2841, -9.7149) centre (-249.0745, 216.5779) ccw
  arc A1553 (-26.0864, -12.3896) -> (-25.3116, -11.7199) centre (-31.04, -5.8754) ccw
  arc A1554 (-26.526, -12.5703) -> (-26.0864, -12.3896) centre (-26.6459, -11.6538) ccw
  arc A1555 (-26.8552, -12.4305) -> (-26.526, -12.5703) centre (-26.5718, -12.2207) ccw
  arc A1556 (-26.9361, -12.0363) -> (-26.8552, -12.4305) centre (-26.4711, -12.1462) ccw
  arc A1557 (-26.7105, -11.5486) -> (-26.9361, -12.0363) centre (-25.6285, -12.3453) ccw
  arc A1558 (-26.0409, -10.7475) -> (-26.7105, -11.5486) centre (-19.8791, -16.5786) ccw
  arc A1559 (-24.1951, -8.8177) -> (-26.0409, -10.7475) centre (157.079, -184.0405) ccw
  arc A1560 (-23.0264, -7.6171) -> (-24.1951, -8.8177) centre (147.4141, -174.6981) ccw
  arc A1561 (-22.0182, -6.6001) -> (-23.0264, -7.6171) centre (68.2784, -97.1222) ccw
  arc A1562 (-21.1267, -5.7129) -> (-22.0182, -6.6001) centre (357.5819, -387.149) ccw
  arc A1563 (-21.0267, -5.6571) -> (-21.1267, -5.7129) centre (-20.9774, -5.8633) ccw
  arc A1564 (-20.946, -5.6691) -> (-21.0267, -5.6571) centre (-21.0012, -5.7635) ccw
  arc A1565 (-20.8042, -5.7629) -> (-20.946, -5.6691) centre (-21.7196, -6.9923) ccw
  arc A1566 (-20.6415, -5.899) -> (-20.8042, -5.7629) centre (-21.9299, -7.2747) ccw
  arc A1567 (-20.4765, -6.0668) -> (-20.6415, -5.899) centre (-22.5901, -7.9796) ccw
  arc A1568 (-17.8542, -8.4653) -> (-17.868, -8.1761) centre (-18.0534, -8.3299) ccw
  arc A1569 (-18.357, -9.1301) -> (-17.8542, -8.4653) centre (-24.671, -3.8324) ccw
  arc A1570 (-19.263, -10.1334) -> (-18.357, -9.1301) centre (-32.5764, 2.8006) ccw
  arc A1571 (-20.9158, -11.8085) -> (-19.263, -10.1334) centre (-128.2476, 95.7445) ccw
  arc A1572 (-23.0023, -13.8721) -> (-20.9158, -11.8085) centre (-251.2376, 218.9886) ccw
  arc A1573 (-23.8163, -14.5792) -> (-23.0023, -13.8721) centre (-29.2873, -7.4597) ccw
  arc A1574 (-24.2924, -14.7978) -> (-23.8163, -14.5792) centre (-24.532, -13.6479) ccw
  arc A1575 (-24.6622, -14.6874) -> (-24.2924, -14.7978) centre (-24.3752, -14.4004) ccw
  arc A1576 (-24.7758, -14.3217) -> (-24.6622, -14.6874) centre (-24.3714, -14.3966) ccw
  arc A1577 (-24.5704, -13.8579) -> (-24.7758, -14.3217) centre (-23.6992, -14.521) ccw
  arc A1578 (-23.8894, -13.07) -> (-24.5704, -13.8579) centre (-17.9033, -18.9323) ccw
  arc A1579 (-21.8975, -11.055) -> (-23.8894, -13.07) centre (193.1222, -225.5976) ccw
  arc A1580 (-20.6524, -9.8276) -> (-21.8975, -11.055) centre (52.8215, -85.608) ccw
  arc A1581 (-19.5579, -8.7935) -> (-20.6524, -9.8276) centre (19.9207, -51.6744) ccw
  arc A1582 (-18.6048, -7.9242) -> (-19.5579, -8.7935) centre (74.3467, -110.7911) ccw
  arc A1583 (-18.4194, -7.8528) -> (-18.6048, -7.9242) centre (-18.4194, -8.1294) ccw
  arc A1584 (-18.2916, -7.8759) -> (-18.4194, -7.8528) centre (-18.4194, -8.2175) ccw
  arc A1585 (-18.1407, -7.9478) -> (-18.2916, -7.8759) centre (-18.6321, -8.7861) ccw
  arc A1586 (-17.9916, -8.0524) -> (-18.1407, -7.9478) centre (-18.705, -8.9104) ccw
  arc A1587 (-17.868, -8.1761) -> (-17.9916, -8.0524) centre (-18.5986, -8.7823) ccw
  arc A1588 (-16.676, -9.4627) -> (-16.762, -9.1542) centre (-16.9178, -9.3638) ccw
  arc A1589 (-16.9799, -9.9803) -> (-16.676, -9.4627) centre (-18.6297, -8.664) ccw
  arc A1590 (-17.7718, -10.8786) -> (-16.9799, -9.9803) centre (-26.508, -2.3783) ccw
  arc A1591 (-19.7115, -12.851) -> (-17.7718, -10.8786) centre (-204.1848, 170.5021) ccw
  arc A1592 (-21.8438, -14.9775) -> (-19.7115, -12.851) centre (-262.6455, 228.6079) ccw
  arc A1593 (-22.6678, -15.6998) -> (-21.8438, -14.9775) centre (-28.2708, -8.4762) ccw
  arc A1594 (-23.1576, -15.9298) -> (-22.6678, -15.6998) centre (-23.4251, -14.7234) ccw
  arc A1595 (-23.5533, -15.8309) -> (-23.1576, -15.9298) centre (-23.2564, -15.4841) ccw
  arc A1596 (-23.6907, -15.4752) -> (-23.5533, -15.8309) centre (-23.2917, -15.5254) ccw
  arc A1597 (-23.5063, -15.0232) -> (-23.6907, -15.4752) centre (-22.7566, -15.5926) ccw
  arc A1598 (-22.8291, -14.2396) -> (-23.5063, -15.0232) centre (-16.9747, -19.9836) ccw
  arc A1599 (-20.7457, -12.1341) -> (-22.8291, -14.2396) centre (226.2685, -258.6399) ccw
  arc A1600 (-19.4769, -10.8729) -> (-20.7457, -12.1341) centre (135.6666, -168.2244) ccw
  arc A1601 (-18.3854, -9.8107) -> (-19.4769, -10.8729) centre (62.3486, -93.863) ccw
  arc A1602 (-17.4173, -8.8831) -> (-18.3854, -9.8107) centre (364.7888, -408.7337) ccw
  arc A1603 (-17.3208, -8.8444) -> (-17.4173, -8.8831) centre (-17.3208, -8.9841) ccw
  arc A1604 (-17.2418, -8.862) -> (-17.3208, -8.8444) centre (-17.3208, -9.0304) ccw
  arc A1605 (-17.0981, -8.9354) -> (-17.2418, -8.862) centre (-18.2494, -11.0117) ccw
  arc A1606 (-16.932, -9.0356) -> (-17.0981, -8.9354) centre (-18.3859, -11.2579) ccw
  arc A1607 (-16.762, -9.1542) -> (-16.932, -9.0356) centre (-18.8274, -11.9328) ccw
  arc A1608 (-15.1299, -10.6619) -> (-15.4014, -10.336) centre (-16.5486, -11.5673) ccw
  arc A1609 (-14.972, -11.0236) -> (-15.1299, -10.6619) centre (-16.199, -11.3442) ccw
  arc A1610 (-14.8972, -11.5192) -> (-14.972, -11.0236) centre (-17.2666, -11.6232) ccw
  arc A1611 (-14.8854, -12.3107) -> (-14.8972, -11.5192) centre (-28.5468, -12.1184) ccw
  arc A1612 (-14.9141, -12.8916) -> (-14.8854, -12.3107) centre (-23.142, -12.1945) ccw
  arc A1613 (-14.9833, -13.417) -> (-14.9141, -12.8916) centre (-20.5972, -12.4101) ccw
  arc A1614 (-15.0778, -13.8381) -> (-14.9833, -13.417) centre (-19.8807, -12.5386) ccw
  arc A1615 (-15.1895, -14.0061) -> (-15.0778, -13.8381) centre (-15.3851, -13.7549) ccw
  arc A1616 (-15.4015, -14.1392) -> (-15.1895, -14.0061) centre (-15.9536, -13.0251) ccw
  arc A1617 (-16.227, -14.5442) -> (-15.4015, -14.1392) centre (-66.8439, 89.6772) ccw
  arc A1618 (-17.2108, -15.0135) -> (-16.227, -14.5442) centre (-50.2504, 55.5108) ccw
  arc A1619 (-18.3235, -15.5281) -> (-17.2108, -15.0135) centre (-70.0028, 97.6729) ccw
  arc A1620 (-18.3235, -15.5281) -> (-19.4451, -16.0417) centre (209.1579, -513.8153) ccw
  arc A1621 (-19.4451, -16.0417) -> (-20.4563, -16.508) centre (132.4227, -346.7287) ccw
  arc A1622 (-20.4563, -16.508) -> (-21.3044, -16.9017) centre (174.0266, -436.5936) ccw
  arc A1623 (-21.3044, -16.9017) -> (-21.5809, -17.0362) centre (-17.5403, -24.9894) ccw
  arc A1624 (-21.782, -17.0992) -> (-21.5809, -17.0362) centre (-21.8687, -16.4695) ccw
  arc A1625 (-22.0019, -17.0969) -> (-21.782, -17.0992) centre (-21.8844, -16.3558) ccw
  arc A1626 (-22.2284, -17.0288) -> (-22.0019, -17.0969) centre (-21.8642, -16.2286) ccw
  arc A1627 (-22.4485, -16.8986) -> (-22.2284, -17.0288) centre (-21.7334, -15.941) ccw
  arc A1628 (-22.5648, -16.5718) -> (-22.4485, -16.8986) centre (-22.2612, -16.6479) ccw
  arc A1629 (-22.3342, -16.0985) -> (-22.5648, -16.5718) centre (-21.3278, -16.8817) ccw
  arc A1630 (-21.6032, -15.2609) -> (-22.3342, -16.0985) centre (-14.525, -22.1757) ccw
  arc A1631 (-19.5664, -13.1952) -> (-21.6032, -15.2609) centre (202.8791, -234.5645) ccw
  arc A1632 (-18.2745, -11.9073) -> (-19.5664, -13.1952) centre (142.3826, -174.3606) ccw
  arc A1633 (-17.1635, -10.8227) -> (-18.2745, -11.9073) centre (66.3597, -97.4877) ccw
  arc A1634 (-16.1777, -9.8749) -> (-17.1635, -10.8227) centre (384.9389, -428.0497) ccw
  arc A1635 (-16.0808, -9.8359) -> (-16.1777, -9.8749) centre (-16.0808, -9.976) ccw
  arc A1636 (-15.9984, -9.8605) -> (-16.0808, -9.8359) centre (-16.0808, -9.9862) ccw
  arc A1637 (-15.8224, -9.9828) -> (-15.9984, -9.8605) centre (-18.1549, -13.1517) ccw
  arc A1638 (-15.6174, -10.1444) -> (-15.8224, -9.9828) centre (-18.1547, -13.1514) ccw
  arc A1639 (-15.4014, -10.336) -> (-15.6174, -10.1444) centre (-19.4063, -14.6347) ccw
  arc A1640 (-38.2398, -8.3061) -> (-38.6683, -9.2385) centre (-36.9718, -9.4536) ccw
  arc A1641 (-38.6683, -9.2385) -> (-38.4666, -10.2141) centre (-37.1435, -9.4319) ccw
  arc A1642 (-38.4666, -10.2141) -> (-37.7066, -10.8671) centre (-37.1243, -9.4205) ccw
  arc A1643 (-37.7066, -10.8671) -> (-36.675, -10.9531) centre (-37.0514, -9.2393) ccw
  arc A1644 (-36.675, -10.9531) -> (-36.1346, -10.7434) centre (-37.08, -9.1091) ccw
  arc A1645 (-36.1346, -10.7434) -> (-35.7421, -10.3931) centre (-36.7843, -9.6203) ccw
  arc A1646 (-35.7421, -10.3931) -> (-35.507, -9.8997) centre (-36.8846, -9.5459) ccw
  arc A1647 (-35.507, -9.8997) -> (-35.4275, -9.2709) centre (-37.9554, -9.2709) ccw
  arc A1648 (-35.4275, -9.2709) -> (-35.7226, -8.4804) centre (-36.634, -9.2709) ccw
  arc A1649 (-35.7226, -8.4804) -> (-36.506, -7.952) centre (-37.0959, -9.6715) ccw
  arc A1650 (-36.506, -7.952) -> (-37.4698, -7.8786) centre (-37.129, -9.7679) ccw
  arc A1651 (-37.4698, -7.8786) -> (-38.2398, -8.3061) centre (-37.2274, -9.2224) ccw
  arc A1652 (-35.7991, -9.2601) -> (-36.0324, -8.7083) centre (-37.432, -9.6253) ccw
  arc A1653 (-35.8057, -9.8083) -> (-35.7991, -9.2601) centre (-36.9617, -9.5201) ccw
  arc A1654 (-36.0521, -10.2638) -> (-35.8057, -9.8083) centre (-36.8149, -9.5567) ccw
  arc A1655 (-36.4936, -10.5586) -> (-36.0521, -10.2638) centre (-36.8899, -9.4872) ccw
  arc A1656 (-37.361, -10.639) -> (-36.4936, -10.5586) centre (-37.0773, -8.9807) ccw
  arc A1657 (-38.0446, -10.2513) -> (-37.361, -10.639) centre (-37.1659, -9.4984) ccw
  arc A1658 (-38.305, -9.5318) -> (-38.0446, -10.2513) centre (-37.2225, -9.5469) ccw
  arc A1659 (-38.0598, -8.7306) -> (-38.305, -9.5318) centre (-36.8049, -9.5528) ccw
  arc A1660 (-37.6006, -8.2743) -> (-38.0598, -8.7306) centre (-36.7525, -9.5872) ccw
  arc A1661 (-37.0432, -8.1066) -> (-37.6006, -8.2743) centre (-37.0317, -9.155) ccw
  arc A1662 (-36.4876, -8.2627) -> (-37.0432, -8.1066) centre (-37.0319, -9.1334) ccw
  arc A1663 (-36.0324, -8.7083) -> (-36.4876, -8.2627) centre (-37.2753, -9.5226) ccw
  arc A1664 (37.3554, -9.2655) -> (38.8139, -8.4818) centre (31.6743, 3.0565) ccw
  arc A1665 (35.9779, -9.7588) -> (37.3554, -9.2655) centre (33.8748, -1.7163) ccw
  arc A1666 (34.471, -10.0222) -> (35.9779, -9.7588) centre (33.6366, -0.8055) ccw
  arc A1667 (32.609, -10.1044) -> (34.471, -10.0222) centre (32.6508, 10.084) ccw
  arc A1668 (32.609, -10.1044) -> (30.7596, -10.1704) centre (32.5582, -34.6217) ccw
  arc A1669 (30.7596, -10.1704) -> (29.8179, -10.4471) centre (30.9304, -12.4921) ccw
  arc A1670 (29.8179, -10.4471) -> (29.2425, -11.0391) centre (30.4827, -11.6691) ccw
  arc A1671 (29.2425, -11.0391) -> (28.8061, -12.1732) centre (34.5261, -13.7232) ccw
  arc A1672 (28.8061, -12.1732) -> (28.6946, -13.1974) centre (32.0023, -13.0393) ccw
  arc A1673 (28.6946, -13.1974) -> (28.9755, -13.9574) centre (30.0367, -13.1333) ccw
  arc A1674 (28.9755, -13.9574) -> (29.7691, -14.661) centre (31.2506, -12.1906) ccw
  arc A1675 (29.7691, -14.661) -> (31.4667, -15.5992) centre (43.9022, 8.906) ccw
  line L88 (31.4667, -15.5992) -> (33.7869, -16.7767)
  line L89 (33.7869, -16.7767) -> (36.7038, -16.7767)
  arc A1676 (36.7038, -16.7767) -> (38.0549, -16.7599) centre (36.7038, 37.5517) ccw
  arc A1677 (38.0549, -16.7599) -> (38.9849, -16.7029) centre (37.7363, -3.9494) ccw
  arc A1678 (38.9849, -16.7029) -> (39.6245, -16.6128) centre (38.2392, -9.0866) ccw
  arc A1679 (39.6245, -16.6128) -> (39.8687, -16.4668) centre (39.5509, -16.2126) ccw
  arc A1680 (39.8687, -16.4668) -> (40.1653, -15.9168) centre (38.5067, -15.3773) ccw
  arc A1681 (40.1653, -15.9168) -> (41.1259, -12.9262) centre (-362.1817, 114.9689) ccw
  arc A1682 (41.1259, -12.9262) -> (42.0519, -9.9617) centre (-301.0481, 95.5818) ccw
  arc A1683 (42.0519, -9.9617) -> (42.1603, -9.2402) centre (39.7062, -9.2402) ccw
  arc A1684 (42.1603, -9.2402) -> (42.0197, -8.7742) centre (41.3178, -9.2402) ccw
  arc A1685 (42.0197, -8.7742) -> (41.6039, -8.313) centre (40.261, -9.9417) ccw
  arc A1686 (41.6039, -8.313) -> (41.0465, -7.9726) centre (40.1296, -10.1011) ccw
  arc A1687 (41.0465, -7.9726) -> (40.4871, -7.8606) centre (40.5027, -9.235) ccw
  arc A1688 (40.4871, -7.8606) -> (40.1568, -7.9057) centre (40.5024, -9.205) ccw
  arc A1689 (40.1568, -7.9057) -> (39.7144, -8.0463) centre (41.4057, -12.6014) ccw
  arc A1690 (39.7144, -8.0463) -> (39.2436, -8.2464) centre (41.633, -13.2134) ccw
  arc A1691 (39.2436, -8.2464) -> (38.8139, -8.4818) centre (41.2534, -12.4243) ccw
  arc A1692 (41.4241, -8.6697) -> (41.275, -8.4902) centre (40.3798, -9.3855) ccw
  arc A1693 (41.5501, -8.8866) -> (41.4241, -8.6697) centre (40.0328, -9.6233) ccw
  arc A1694 (41.6366, -9.1063) -> (41.5501, -8.8866) centre (40.17, -9.5567) ccw
  arc A1695 (41.6646, -9.2925) -> (41.6366, -9.1063) centre (41.0301, -9.2925) ccw
  arc A1696 (41.5675, -9.5551) -> (41.6646, -9.2925) centre (41.2608, -9.2925) ccw
  arc A1697 (40.7008, -10.5499) -> (41.5675, -9.5551) centre (-16.5491, 40.2095) ccw
  arc A1698 (39.6409, -11.7032) -> (40.7008, -10.5499) centre (7.7312, 18.6819) ccw
  arc A1699 (38.3835, -12.9931) -> (39.6409, -11.7032) centre (-16.0145, 41.293) ccw
  arc A1700 (38.3835, -12.9931) -> (37.1433, -14.2543) centre (123.3258, -97.7606) ccw
  arc A1701 (37.1433, -14.2543) -> (36.142, -15.3151) centre (77.2845, -53.1491) ccw
  arc A1702 (36.142, -15.3151) -> (35.3281, -16.2088) centre (128.251, -100.017) ccw
  arc A1703 (35.3281, -16.2088) -> (35.3601, -16.2809) centre (35.3601, -16.2377) ccw
  arc A1704 (35.3601, -16.2809) -> (35.5286, -16.2156) centre (35.3601, -16.031) ccw
  arc A1705 (35.5286, -16.2156) -> (36.3938, -15.4186) centre (-49.5554, 77.0148) ccw
  arc A1706 (36.3938, -15.4186) -> (37.3873, -14.4705) centre (0.3208, 23.376) ccw
  arc A1707 (37.3873, -14.4705) -> (38.5172, -13.3453) centre (-29.7973, 54.1278) ccw
  arc A1708 (39.6293, -12.2301) -> (38.5172, -13.3453) centre (155.0926, -128.4849) ccw
  arc A1709 (40.565, -11.3162) -> (39.6293, -12.2301) centre (94.8869, -67.8665) ccw
  arc A1710 (41.3742, -10.5419) -> (40.565, -11.3162) centre (235.5146, -214.2635) ccw
  arc A1711 (41.4167, -10.5601) -> (41.3742, -10.5419) centre (41.3916, -10.5601) ccw
  arc A1712 (41.4009, -10.663) -> (41.4167, -10.5601) centre (41.073, -10.5601) ccw
  arc A1713 (41.2835, -11.0294) -> (41.4009, -10.663) centre (10.5059, -0.9643) ccw
  arc A1714 (41.137, -11.462) -> (41.2835, -11.0294) centre (20.5036, -4.2338) ccw
  arc A1715 (40.9633, -11.9464) -> (41.137, -11.462) centre (7.9333, 0.1698) ccw
  arc A1716 (40.6631, -12.5999) -> (40.9633, -11.9464) centre (36.6901, -10.3789) ccw
  arc A1717 (40.2413, -13.2552) -> (40.6631, -12.5999) centre (35.1917, -9.5413) ccw
  arc A1718 (39.6712, -13.9504) -> (40.2413, -13.2552) centre (33.3637, -8.1968) ccw
  arc A1719 (38.9183, -14.7269) -> (39.6712, -13.9504) centre (26.5489, -1.9805) ccw
  arc A1720 (38.9183, -14.7269) -> (38.327, -15.3201) centre (56.5154, -32.8605) ccw
  arc A1721 (38.327, -15.3201) -> (37.8752, -15.8192) centre (45.9957, -22.7156) ccw
  arc A1722 (37.8752, -15.8192) -> (37.567, -16.2033) centre (44.5813, -21.5144) ccw
  arc A1723 (37.567, -16.2033) -> (37.6025, -16.2762) centre (37.6033, -16.2308) ccw
  arc A1724 (37.6025, -16.2762) -> (37.7634, -16.2224) centre (37.6068, -16.0218) ccw